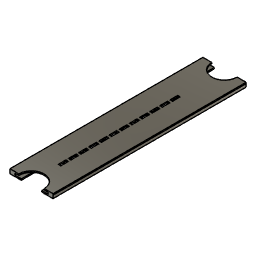
Slide_holder (Autodesk Fusion 360 design; units mm, degrees)
Autodesk Fusion 360 part; units mm, degrees
sketch "Sketch1" plane through (0, 0, 0) normal (0, 0, 1) x (1, 0, 0)
  line L0 (-17, 0) -> (16.96, 0)
  line L1 (16.96, 0) -> (16.96, 151.9)
  line L2 (16.96, 151.9) -> (-17, 151.9)
  line L3 (-17, 151.9) -> (-17, 0)
  line L4 (-8.02, 0) -> (7.98, 0)
  line L5 (7.98, 0) -> (7.98, 151.9)
  line L6 (7.98, 151.9) -> (-8.02, 151.9)
  line L7 (-8.02, 151.9) -> (-8.02, 0)
  dimension "d1" = 33.96
  dimension "d2" = 151.9
  dimension "d7" = 16
  dimension "d8" = 151.9
  dimension "d9" = 8.98
  constraint horizontal L0
  constraint vertical L1
  constraint horizontal L2
  constraint vertical L3
  constraint horizontal L4
  constraint vertical L5
  constraint horizontal L6
  constraint vertical L7
  constraint coincident L0 L4.start
  measures "d1" distance of L0.start L0.end
  measures "d2" distance of L0.start L2.end
  measures "d7" distance of L4.start L4.end
  measures "d8" distance of L4.start L6.end
  measures "d9" distance of L1 L5
extrude "Extrude1" add sketch "Sketch1" along normal blind 1 contours L0 L2 L3 L7 | L0 L1 L2 L5 makes body 1 at (-14.0067, 50.6333, 0) makes body 2 at (10.9733, 101.2667, 0)
sketch "Sketch2" plane through (0, 0, 1) normal (0, 0, 1) x (-1, 0, 0)
  line L0 (8.02, -151.9) -> (17, -151.9)
  line L1 (17, -151.9) -> (17, 0)
  line L2 (17, 0) -> (8.02, 0)
  line L3 (8.02, 0) -> (8.02, -151.9)
  line L4 (17, 0) -> (13.04, 0)
  line L5 (13.04, 0) -> (13.04, -151.9)
  line L6 (13.04, -151.9) -> (17, -151.9)
  line L7 (17, -151.9) -> (17, 0)
  line L8 (-16.96, 0) -> (-13, 0)
  line L9 (-13, 0) -> (-13, -151.9)
  line L10 (-13, -151.9) -> (-16.96, -151.9)
  line L11 (-16.96, -151.9) -> (-16.96, 0)
  line L12 (-16.96, 0) -> (-16.96, -151.9)
  line L13 (-16.96, -151.9) -> (-7.98, -151.9)
  line L14 (-7.98, -151.9) -> (-7.98, 0)
  line L15 (-7.98, 0) -> (-16.96, 0)
  dimension "d10" = 3.96
  dimension "d11" = 3.96
  dimension "d24" = 151.9
  dimension "d25" = 151.9
  constraint horizontal L4
  constraint vertical L5
  constraint horizontal L6
  constraint vertical L7
  constraint coincident L1.end L2.start
  constraint horizontal L8
  constraint vertical L9
  constraint horizontal L10
  constraint vertical L11
  constraint collinear L11 L12
  measures "d10" distance of L1.end L4.end
  measures "d11" distance of L8.start L8.end
  measures "d24" distance of L1.end L0.end
  measures "d25" distance of L8.start L10.end
extrude "Extrude2" add sketch "Sketch2" along normal blind 1.4 contours L0 L1 L2 L4 L5 L6 L7 | L8 L9 L10 L11 L12 L13 L15 bodies 1 2
sketch "Sketch3" plane through (0, 0, 2.4) normal (0, 0, 1) x (-1, 0, 0)
  line L0 (13.04, -151.9) -> (17, -151.9)
  line L1 (17, -151.9) -> (17, 0)
  line L2 (17, 0) -> (13.04, 0)
  line L3 (13.04, 0) -> (13.04, -151.9)
  line L4 (17, 0) -> (13.04, 0)
  line L5 (13.04, 0) -> (13.04, -151.9)
  line L6 (13.04, -151.9) -> (17, -151.9)
  line L7 (17, -151.9) -> (17, 0)
  line L8 (17, -151.9) -> (-17, -151.9)
  line L9 (-17, -151.9) -> (-17, 0)
  line L10 (-17, 0) -> (17, 0)
  line L11 (17, 0) -> (17, -151.9)
  line L12 (0.98, -28) -> (-1.02, -28)
  line L13 (-1.02, -28) -> (-1.02, -22)
  line L14 (-1.02, -22) -> (0.98, -22)
  line L15 (0.98, -22) -> (0.98, -28)
  line L16 (-1.02, -30) -> (0.98, -30)
  line L17 (0.98, -30) -> (0.98, -36)
  line L18 (0.98, -36) -> (-1.02, -36)
  line L19 (-1.02, -36) -> (-1.02, -30)
  line L20 (-1.02, -38) -> (0.98, -38)
  line L21 (0.98, -38) -> (0.98, -44)
  line L22 (0.98, -44) -> (-1.02, -44)
  line L23 (-1.02, -44) -> (-1.02, -38)
  line L24 (-1.02, -46) -> (0.98, -46)
  line L25 (0.98, -46) -> (0.98, -52)
  line L26 (0.98, -52) -> (-1.02, -52)
  line L27 (-1.02, -52) -> (-1.02, -46)
  line L28 (-1.02, -54) -> (0.98, -54)
  line L29 (0.98, -54) -> (0.98, -60)
  line L30 (0.98, -60) -> (-1.02, -60)
  line L31 (-1.02, -60) -> (-1.02, -54)
  line L32 (-1.02, -62) -> (0.98, -62)
  line L33 (0.98, -62) -> (0.98, -68)
  line L34 (0.98, -68) -> (-1.02, -68)
  line L35 (-1.02, -68) -> (-1.02, -62)
  line L36 (-1.02, -70) -> (0.98, -70)
  line L37 (0.98, -70) -> (0.98, -76)
  line L38 (0.98, -76) -> (-1.02, -76)
  line L39 (-1.02, -76) -> (-1.02, -70)
  line L40 (-1.02, -78) -> (0.98, -78)
  line L41 (0.98, -78) -> (0.98, -84)
  line L42 (0.98, -84) -> (-1.02, -84)
  line L43 (-1.02, -84) -> (-1.02, -78)
  line L44 (-1.02, -86) -> (0.98, -86)
  line L45 (0.98, -86) -> (0.98, -92)
  line L46 (0.98, -92) -> (-1.02, -92)
  line L47 (-1.02, -92) -> (-1.02, -86)
  line L48 (-1.02, -94) -> (0.98, -94)
  line L49 (0.98, -94) -> (0.98, -100)
  line L50 (0.98, -100) -> (-1.02, -100)
  line L51 (-1.02, -100) -> (-1.02, -94)
  line L52 (-1.02, -102) -> (0.98, -102)
  line L53 (0.98, -102) -> (0.98, -108)
  line L54 (0.98, -108) -> (-1.02, -108)
  line L55 (-1.02, -108) -> (-1.02, -102)
  line L56 (-1.02, -110) -> (0.98, -110)
  line L57 (0.98, -110) -> (0.98, -116)
  line L58 (0.98, -116) -> (-1.02, -116)
  line L59 (-1.02, -116) -> (-1.02, -110)
  arc A0 (10, -151.9) -> (-10, -151.9) centre (0, -151.9) ccw
  arc A1 (-10.02, 0) -> (9.98, 0) centre (-0.02, 0) ccw
  dimension "d26" = 34
  dimension "d27" = 151.9
  dimension "d29" = 2
  dimension "d30" = 6
  dimension "d31" = 22
  dimension "d32" = 15.98
  dimension "d35" = 0
  dimension "d36" = -8
  dimension "d37" = 20
  dimension "d38" = 17
  dimension "d40" = 20
  dimension "d41" = 16.98
  constraint horizontal L4
  constraint vertical L5
  constraint horizontal L6
  constraint vertical L7
  constraint coincident L0.start L3.end
  constraint coincident L1.end L2.start
  constraint horizontal L8
  constraint vertical L9
  constraint horizontal L10
  constraint vertical L11
  constraint coincident L0.end L1.start
  constraint horizontal L12
  constraint vertical L13
  constraint horizontal L14
  constraint vertical L15
  constraint coincident L8 A0.start
  constraint coincident L8 A0.end
  constraint coincident L10 A1.end
  constraint coincident L10 A1.start
  constraint coincident L10 A1.centre
  constraint coincident L8 A0.centre
  measures "d26" distance of L0.end L8.end
  measures "d27" distance of L0.end L1.end
  measures "d29" distance of L12.start L12.end
  measures "d30" distance of L12.start L14.end
  measures "d31" distance of L10 L14
  measures "d32" distance of L9 L13
  measures "d37" distance of A0.end A0.start
  measures "d38" distance of L11 A0.centre
  measures "d40" distance of A1.start A1.end
  measures "d41" distance of L9 A1.centre
extrude "Extrude3" add sketch "Sketch3" along normal blind 1 contours L0 L1 L2 L3 L4 L5 L6 L7 L8 L10 L11 | L3 L5 L8 L9 L10 A0 A1 bodies 1 2
